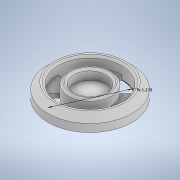
# Autodesk Inventor part: Dowel_Tube_Mount
Saved by Autodesk Inventor 2020.2 (Build 242310000, 310)
## iProperties
Created: 2020-03-07
Part Number: Dowel_Tube_Mount
Material: Generic
Document SubType Name: Modeling
Designer: antho
Density: 1 g/cm^3
Appearance: Default
Author: antho
Autodesk Inventor part; units mm, degrees
ref_plane "YZ Plane" through (0, 0, 0) normal (1, 0, 0) x (0, 1, 0)
ref_plane "XZ Plane" through (0, 0, 0) normal (0, 1, 0) x (-1, 0, 0)
ref_plane "XY Plane" through (0, 0, 0) normal (0, 0, 1) x (1, 0, 0)
sketch "Sketch1" plane through (0, 0, 0) normal (0, 1, 0) x (-1, 0, 0)
  circle A0 centre (0, 0) radius 15.621
  circle A1 centre (0, 0) radius 7.9375
  circle A2 centre (0, 0) radius 10.4375
  circle A3 centre (0, 0) radius 20.621
  dimension "TubeDiameter" = 31.242
  dimension "RodDiameter" = 15.875
  dimension "RodGuardDiameter" = 20.875
  dimension "HiltGuardDiameter" = 41.242
  constraints: 4 centre point, 4 coincident
  measures "TubeDiameter" diameter of A0
  measures "RodDiameter" diameter of A1
  measures "RodGuardDiameter" diameter of A2
  measures "HiltGuardDiameter" diameter of A3
extrude "Tube&DowelMount" add sketch "Sketch1" along normal blind 5
sketch "Sketch23" plane through (0, 0, 0) normal (0, -1, 0) x (1, 0, 0)
  circle A0 centre (0, 0) radius 20.621
  line L0 (0, 0) -> (0, -20.621)
  circle A1 centre (0, 0) radius 20.621 projected
  circle A2 centre (0, 0) radius 10.4375
  circle A3 centre (0, 0) radius 15.621
  line L1 (0, 0) -> (14.5812, -14.5812)
  line L2 (0, 0) -> (20.621, 0)
  line L3 (0, 0) -> (14.5812, 14.5812)
  line L4 (0, 0) -> (0, 20.621)
  line L5 (0, 0) -> (-14.5812, 14.5812)
  line L6 (0, 0) -> (-20.621, 0)
  line L7 (0, 0) -> (-14.5812, -14.5812)
  point P0 (0, -15.621)
  point P1 (0, -10.4375)
  point P2 (7.3804, -7.3804)
  point P3 (11.0457, -11.0457)
  point P4 (-11.0457, -11.0457)
  point P5 (-15.621, 0)
  point P6 (-10.4375, 0)
  point P7 (-7.3804, -7.3804)
  point P8 (10.4375, 0)
  point P9 (7.3804, 7.3804)
  point P10 (11.0457, 11.0457)
  point P11 (15.621, 0)
  point P12 (0, 10.4375)
  point P13 (-7.3804, 7.3804)
  point P14 (-11.0457, 11.0457)
  point P15 (0, 15.621)
  dimension "d128" = 41.242
  dimension "d129" = 20.875
  dimension "d130" = 31.242
  dimension "d133" = 360
  constraints: 16 end point, 3 centre point, 3 coincident, 1 vertical, 1 vertical alignment, 26 other
  measures "d128" diameter of A0
  measures "d129" diameter of A2
  measures "d130" diameter of A3
extrude "WireHole" add sketch "Sketch23" along normal blind 2 contours L2 A3 L3 A0 | A0 L1 A3 L2 | L3 A3 L4 A0 | A0 L0 A3 L1 | A3 L1 A2 L2 | L4 A3 L5 A0 | L3 A2 L4 A3 | A0 L7 A3 L0 | L2 L3 A2 | A2 L1 L2 | L5 A3 L6 A0 | L3 L4 A2 | A0 L6 A3 L7 | A3 L7 A2 L0 | A2 L0 L1 | L5 A2 L4 | L6 A2 L5 | L7 A2 L6 | L0 A2 L7 | L5 A2 L6 A3
sketch "Sketch25" plane through (0, -2, 0) normal (0, -1, 0) x (1, 0, 0)
  circle A0 centre (0, 0) radius 15.621
  dimension "d138" = 31.242
  constraints: 1 centre point, 1 coincident
  measures "d138" diameter of A0
chamfer "Chamfer1" distance 3.175 angle 45 1 edges at (20.621, 5, 0)
chamfer "Chamfer2" distance 1 angle 45 2 edges at (10.4375, 5, 0) (7.9375, 5, 0)
chamfer "Chamfer3" distance 1 angle 45 1 edges at (15.621, 5, 0)
equation "\"Clearance_1\" = 5"
body "Solid1"
